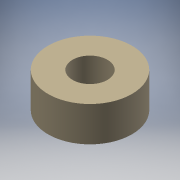
# Autodesk Inventor part: В.шарн. - ось
Saved by Autodesk Inventor 2018 (Build 220112000, 112)
## iProperties
Created: 2020-02-22
Part Number: В.шарн. - ось
Material: Типовые
Document SubType Name: Modeling
Designer: Leancher
Density: 1 g/cm^3
Appearance: По умолчанию
Author: Leancher
Autodesk Inventor part; units mm, degrees
ref_plane "YZ Plane" through (0, 0, 0) normal (1, 0, 0) x (0, 1, 0)
ref_plane "XZ Plane" through (0, 0, 0) normal (0, 1, 0) x (-1, 0, 0)
ref_plane "XY Plane" through (0, 0, 0) normal (0, 0, 1) x (1, 0, 0)
sketch "Эскиз1" plane through (0, 0, 0) normal (0, 0, 1) x (1, 0, 0)
  circle A0 centre (6.8722, 8.4755) radius 6
  circle A1 centre (6.8722, 8.4755) radius 2.5
  point P0 (0, 0)
  dimension "d5" = 5
  dimension "d6" = 12
  constraints: 2 centre point, 1 coincident
  measures "d5" diameter of A1
  measures "d6" diameter of A0
extrude "Выдавливание1" add sketch "Эскиз1" against normal blind 5
